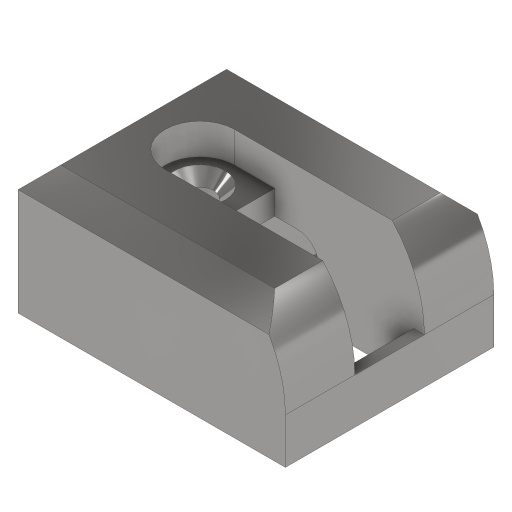
# Autodesk Inventor part: Part015. Fixing Block
Saved by Autodesk Inventor 2023.2 (Build 272271030, 271C)
## iProperties
Created: 2023-09-19
Part Number: Part015. Fixing Block
Material: Steel, Carbon
Document SubType Name: Modeling
Designer: User
Mass: 196.194 g
Surface Area: 90.4387 cm^2
Volume: 24.9928 cm^3
Density: 7.85 g/cm^3
Appearance: Steel - Polished
Author: User
Autodesk Inventor part; units mm, degrees
ref_plane "YZ Plane" through (0, 0, 0) normal (1, 0, 0) x (0, 1, 0)
ref_plane "XZ Plane" through (0, 0, 0) normal (0, 1, 0) x (-1, 0, 0)
ref_plane "XY Plane" through (0, 0, 0) normal (0, 0, 1) x (1, 0, 0)
sketch "Sketch1" plane through (0, 0, 0) normal (0, 0, 1) x (1, 0, 0)
  line L0 (0, 0) -> (50, 0)
  line L1 (50, 0) -> (50, 8.5)
  arc A0 (50, 8.5) -> (43.9926, 24) centre (27, 8.5) ccw
  line L2 (43.9926, 24) -> (0, 24)
  line L3 (0, 24) -> (0, 0)
  dimension "d0" = 50
  dimension "d1" = 24
  dimension "d2" = 8.5
  dimension "d3" = 23
  constraints: 8 end point, 3 perpendicular, 2 point on circle, 1 centre point, 1 horizontal, 1 tangent
  measures "d0" distance of L0.start L0.end
  measures "d1" distance between parallel lines of L0 L2
  measures "d2" distance of L0.end L1.end
  measures "d3" radius of A0
extrude "Extrusion1" add sketch "Sketch1" along normal mid plane 39
sketch "Sketch2" plane through (0, 0, 0) normal (0, 0, 1) x (1, 0, 0)
  line L0 (0, 0) -> (0, 24) projected
  line L1 (0, 13.7) -> (26.2545, 13.7)
  arc A0 (26.2545, 5.7) -> (26.2545, 13.7) centre (26.2545, 9.7) ccw
  line L2 (26.2545, 5.7) -> (24, 5.7)
  line L3 (24, 5.7) -> (24, 0)
  line L4 (50, 0) -> (0, 0) projected
  line L5 (24, 0) -> (0, 0)
  line L6 (0, 0) -> (0, 13.7)
  line L7 (50, 8.5) -> (50, 0) projected
  dimension "d6" = 4
  dimension "d7" = 5.7
  dimension "d8" = 26
  constraints: 10 end point, 2 perpendicular, 2 point on circle, 2 tangent, 1 centre point, 1 collinear, 1 horizontal, 1 parallel, 1 point on line
  measures "d6" radius of A0
  measures "d7" distance between parallel lines of L4 L2
  measures "d8" distance between parallel lines of L7 L3
extrude "Extrusion2" cut sketch "Sketch2" along normal mid plane 31
sketch "Sketch3" plane through (0, 0, 0) normal (0, 0, 1) x (1, 0, 0)
  line L0 (14.5, 24.0258) -> (14.5, 18.2)
  line L1 (14.5, 18.2) -> (22, 18.2)
  line L2 (22, 18.2) -> (22, 0)
  line L3 (0, 13.7) -> (26.2545, 13.7) projected
  line L4 (22, 0) -> (45, 0)
  line L5 (50, 0) -> (0, 0) projected
  line L6 (50, 8.5) -> (50, 0) projected
  line L7 (50, 8.5) -> (50, 24.0258)
  line L8 (50, 24.0258) -> (14.5, 24.0258)
  line L9 (0, 24) -> (43.9926, 24) projected
  line L10 (45, 0) -> (48, 8.5)
  line L11 (48, 8.5) -> (50, 8.5)
  dimension "d11" = 2
  dimension "d12" = 5
  dimension "d13" = 8.5
  dimension "d14" = 4.5
  dimension "d15" = 35.5
  dimension "d16" = 28
  constraints: 16 end point, 2 perpendicular, 2 point on line, 2 vertical, 1 horizontal, 1 parallel
  measures "d11" distance of L10.end L7.start
  measures "d12" distance from line of L6 L4.end
  measures "d13" distance between parallel lines of L5 L11
  measures "d14" distance between parallel lines of L3 L1
  measures "d15" distance between parallel lines of L7 L0
  measures "d16" distance between parallel lines of L7 L2
extrude "Extrusion3" cut sketch "Sketch3" along normal mid plane 13 contours L8 L7 L11 L10 L4 L2 L1 L0
sketch "Sketch4" plane through (0, 24, -19.5) normal (0, 1, 0) x (1, 0, 0)
  line L0 (14.5, -26) -> (14.5, -13) projected
  line L1 (14.5, -13) -> (14.5, -26) projected
  arc A0 (14.5, -13) -> (14.5, -26) centre (14.5, -19.5) ccw
  point P0 (0, -19.5)
  constraints: 2 point on circle, 1 centre point, 1 midpoint
extrude "Extrusion4" cut sketch "Sketch4" against normal up to surface (5.8 mm away)
sketch "Sketch5" plane through (22, 18.2, 6.5) normal (0, 1, 0) x (1, 0, 0)
  arc A0 (-7.5, 13) -> (-7.5, 0) centre (-7.5, 6.5) ccw projected
  point P0 (-22, 6.5)
hole "Hole1" at (14.5, 18.2, 0) direction (0, -1, 0) diameter 5.2 end through all countersink diameter 9.5 countersink angle 90
chamfer "Chamfer1" distance 4 angle 45 3 edges at (21.9963, 24, 19.5) (0, 24, 0) (21.9963, 24, -19.5)
body "Solid1"
